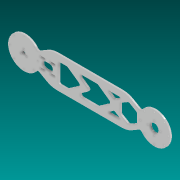
# Autodesk Inventor part: arm1v2
Saved by Autodesk Inventor 2020.3 (Build 243373000, 373)
## iProperties
Created: 2020-05-23
Part Number: arm1v2
Material: Aluminum 6061
Document SubType Name: Sheet Metal
Designer: Svend
Mass: 232.394 g
Surface Area: 513.63 cm^2
Volume: 86.0718 cm^3
Density: 2.7 g/cm^3
Sheet Metal Rule: Default_mm
Appearance: Aluminum - Polished
Author: Svend
Autodesk Inventor part; units mm, degrees
ref_plane "YZ Plane" through (0, 0, 0) normal (1, 0, 0) x (0, 1, 0)
ref_plane "XZ Plane" through (0, 0, 0) normal (0, 1, 0) x (-1, 0, 0)
ref_plane "XY Plane" through (0, 0, 0) normal (0, 0, 1) x (1, 0, 0)
sketch "Sketch1" plane through (0, 0, 0) normal (0, 0, 1) x (1, 0, 0)
  circle A0 centre (346.3464, 0) radius 1.55
  circle A1 centre (330.346, 0) radius 11
  arc A2 (52.2721, 10.7279) -> (52.2721, 14.7279) centre (52.2721, 12.7279) ccw
  line L0 (52.2721, 10.7279) -> (42.2721, 10.7279)
  arc A3 (42.2721, 14.7279) -> (42.2721, 10.7279) centre (42.2721, 12.7279) ccw
  line L1 (42.2721, 14.7279) -> (52.2721, 14.7279)
  arc A4 (77.7279, 10.7279) -> (77.7279, 14.7279) centre (77.7279, 12.7279) ccw
  line L2 (77.7279, 10.7279) -> (67.7279, 10.7279)
  arc A5 (67.7279, 14.7279) -> (67.7279, 10.7279) centre (67.7279, 12.7279) ccw
  line L3 (67.7279, 14.7279) -> (77.7279, 14.7279)
  arc A6 (52.2721, -14.7279) -> (52.2721, -10.7279) centre (52.2721, -12.7279) ccw
  line L4 (52.2721, -14.7279) -> (42.2721, -14.7279)
  arc A7 (42.2721, -10.7279) -> (42.2721, -14.7279) centre (42.2721, -12.7279) ccw
  line L5 (42.2721, -10.7279) -> (52.2721, -10.7279)
  arc A8 (67.7279, -10.7279) -> (67.7279, -14.7279) centre (67.7279, -12.7279) ccw
  line L6 (67.7279, -10.7279) -> (77.7279, -10.7279)
  arc A9 (77.7279, -14.7279) -> (77.7279, -10.7279) centre (77.7279, -12.7279) ccw
  line L7 (77.7279, -14.7279) -> (67.7279, -14.7279)
  circle A10 centre (60, 0) radius 8.5
  circle A11 centre (28, 0) radius 0.5
  line L8 (0, -40) -> (330.346, -40)
  arc A12 (330.346, -40) -> (330.346, 40) centre (330.346, 0) ccw
  line L9 (330.346, 40) -> (0, 40)
  arc A13 (0, 40) -> (0, -40) centre (0, 0) ccw
  line L10 (-4.8, -1) -> (-4.8, 1)
  line L11 (-4.8, 1) -> (-3.873, 1)
  arc A14 (-3.873, -1) -> (-3.873, 1) centre (0, 0) ccw
  line L12 (-3.873, -1) -> (-4.8, -1)
  circle A15 centre (0, 8) radius 2
  circle A16 centre (-6.9282, -4) radius 2
  circle A17 centre (6.9282, -4) radius 2
  circle A18 centre (19.799, 19.799) radius 0.5
  circle A19 centre (0, 28) radius 0.5
  circle A20 centre (-19.799, 19.799) radius 0.5
  circle A21 centre (-28, 0) radius 0.5
  circle A22 centre (-19.799, -19.799) radius 0.5
  circle A23 centre (0, -28) radius 0.5
  circle A24 centre (19.799, -19.799) radius 0.5
  circle A25 centre (330.346, 16.0004) radius 1.55
  circle A26 centre (314.3456, 0) radius 1.55
  circle A27 centre (330.346, -16.0004) radius 1.55
  line L13 (55, 0) -> (65, 0) construction
  line L14 (55, -8.5) -> (65, -8.5)
  line L15 (65, 8.5) -> (55, 8.5)
  arc A28 (55, 8.5) -> (55, -8.5) centre (55, 0) ccw
  arc A29 (65, -8.5) -> (65, 8.5) centre (65, 0) ccw
  point P0 (-4.8, 0)
  point P1 (4, 0)
  point P2 (370.346, 0)
  dimension "d0" = 4
  dimension "d1" = 8.8
  dimension "d2" = 2
  dimension "d6" = 4
  dimension "d7" = 8
  dimension "d14" = 360
  dimension "d16" = 28
  dimension "d17" = 1
  dimension "d20" = 360
  dimension "d22" = 17
  dimension "d23" = 60
  dimension "d24" = 2
  dimension "d25" = 10
  dimension "d26" = 12.7279
  dimension "d27" = 17.7279
  dimension "d28" = 12.7279
  dimension "d29" = 17.7279
  dimension "d30" = 17.7279
  dimension "d31" = 17.7279
  dimension "d32" = 22
  dimension "d33" = 39.9999
  dimension "d35" = 3.1
  dimension "d36" = 16.0004
  dimension "d39" = 360
  dimension "d72" = 270.346
  dimension "d87" = 5
  measures "d0" radius of A14
  measures "d1" distance from line of point (4, 0) L10
  measures "d2" distance between parallel lines of L12 L11
  measures "d6" diameter of A15
  measures "d7" distance of A14.centre A15.centre
  measures "d16" distance of A14.centre A11.centre
  measures "d17" diameter of A11
  measures "d22" diameter of A10
  measures "d23" distance of A14.centre A10.centre
  measures "d24" radius of A3
  measures "d25" distance of L0.start L0.end
  measures "d26" vertical distance of A10.centre A2.centre
  measures "d27" horizontal distance of A10.centre A3.centre
  measures "d28" vertical distance of A8.centre A10.centre
  measures "d29" horizontal distance of A9.centre A10.centre
  measures "d30" horizontal distance of A7.centre A10.centre
  measures "d31" horizontal distance of A4.centre A10.centre
  measures "d32" diameter of A1
  measures "d33" radius of A13
  measures "d35" diameter of A0
  measures "d36" distance of A1.centre A0.centre
  measures "d72" distance of A1.centre A10.centre
  measures "d87" distance of A10.centre L13.end
extrude "Plate1" add sketch "Sketch1" along normal mid plane 4 contours A11 | A13 L9 A12 L8 | A18 | A19 | A20 | A21 | A22 | A23 | A24
sketch "Sketch2" plane through (0, 0, -2) normal (0, 0, -1) x (-1, 0, 0)
  circle A0 centre (-330.346, 0) radius 11 projected
  line L0 (-77.7279, -10.7279) -> (-67.7279, -10.7279) projected
  arc A1 (-67.7279, -14.7279) -> (-67.7279, -10.7279) centre (-67.7279, -12.7279) ccw projected
  line L1 (-67.7279, -14.7279) -> (-77.7279, -14.7279) projected
  arc A2 (-77.7279, -10.7279) -> (-77.7279, -14.7279) centre (-77.7279, -12.7279) ccw projected
  line L2 (-42.2721, -14.7279) -> (-52.2721, -14.7279) projected
  arc A3 (-52.2721, -10.7279) -> (-52.2721, -14.7279) centre (-52.2721, -12.7279) ccw projected
  line L3 (-52.2721, -10.7279) -> (-42.2721, -10.7279) projected
  arc A4 (-42.2721, -14.7279) -> (-42.2721, -10.7279) centre (-42.2721, -12.7279) ccw projected
  line L4 (-67.7279, 10.7279) -> (-77.7279, 10.7279) projected
  arc A5 (-77.7279, 14.7279) -> (-77.7279, 10.7279) centre (-77.7279, 12.7279) ccw projected
  line L5 (-77.7279, 14.7279) -> (-67.7279, 14.7279) projected
  arc A6 (-67.7279, 10.7279) -> (-67.7279, 14.7279) centre (-67.7279, 12.7279) ccw projected
  line L6 (-42.2721, 10.7279) -> (-52.2721, 10.7279) projected
  arc A7 (-52.2721, 14.7279) -> (-52.2721, 10.7279) centre (-52.2721, 12.7279) ccw projected
  line L7 (-52.2721, 14.7279) -> (-42.2721, 14.7279) projected
  arc A8 (-42.2721, 10.7279) -> (-42.2721, 14.7279) centre (-42.2721, 12.7279) ccw projected
  line L8 (3.873, 1) -> (4.8, 1) projected
  line L9 (4.8, 1) -> (4.8, -1) projected
  line L10 (4.8, -1) -> (3.873, -1) projected
  arc A9 (3.873, 1) -> (3.873, -1) centre (0, 0) ccw projected
  circle A10 centre (-6.9282, -4) radius 2 projected
  circle A11 centre (6.9282, -4) radius 2 projected
  circle A12 centre (0, 8) radius 2 projected
  circle A13 centre (-330.346, -16.0004) radius 1.55 projected
  circle A14 centre (-314.3456, 0) radius 1.55 projected
  circle A15 centre (-330.346, 16.0004) radius 1.55 projected
  circle A16 centre (-346.3464, 0) radius 1.55 projected
  line L11 (0, -40) -> (-330.346, -40) projected
  arc A17 (0, -40) -> (0, 40) centre (0, 0) ccw projected
  line L12 (-330.346, 40) -> (0, 40) projected
  arc A18 (-330.346, 40) -> (-330.346, -40) centre (-330.346, 0) ccw projected
  line L13 (-330.346, 40) -> (0, 40) projected
  arc A19 (-330.346, 40) -> (-330.346, -40) centre (-330.346, 0) ccw projected
  line L14 (-330.346, 0) -> (0, 0)
  line L15 (0, -40) -> (-330.346, -40) projected
  line L16 (-210.2693, -25) -> (-250.2693, -25)
  line L17 (-250.2693, -25) -> (-228.346, -12.3426)
  line L18 (-228.346, -12.3426) -> (-210.2693, -25)
  line L19 (-261.064, -40) -> (-295.705, -20)
  line L20 (-222.346, 0) -> (-186.6423, -25)
  line L21 (-186.6423, -25) -> (-131.6423, -25)
  line L22 (-131.6423, -25) -> (-167.346, 0)
  line L23 (-109.6423, -25) -> (-145.346, 0)
  line L24 (-87.346, -25) -> (-109.6423, -25)
  line L25 (-87.346, -25) -> (-87.346, 0)
  line L26 (-210.2693, 25) -> (-250.2693, 25)
  line L27 (-250.2693, 25) -> (-228.346, 12.3426)
  line L28 (-228.346, 12.3426) -> (-210.2693, 25)
  line L29 (-222.346, 0) -> (-186.6423, 25)
  line L30 (-186.6423, 25) -> (-131.6423, 25)
  line L31 (-131.6423, 25) -> (-167.346, 0)
  line L32 (-109.6423, 25) -> (-145.346, 0)
  line L33 (-87.346, 25) -> (-109.6423, 25)
  line L34 (-87.346, 25) -> (-87.346, 0)
  line L35 (-295.705, 20) -> (-261.064, 40)
  line L36 (-261.064, 40) -> (-330.346, 40)
  arc A20 (-295.705, 20) -> (-330.346, 40) centre (-330.346, 0) ccw
  arc A21 (-330.346, -40) -> (-295.705, -20) centre (-330.346, 0) ccw
  line L37 (-286.9966, -12.5) -> (-286.9966, 12.5)
  line L38 (-286.9966, 12.5) -> (-265.346, 25)
  line L39 (-265.346, 25) -> (-243.6954, 12.5)
  line L40 (-243.6954, 12.5) -> (-243.6954, -12.5)
  line L41 (-243.6954, -12.5) -> (-265.346, -25)
  line L42 (-265.346, -25) -> (-286.9966, -12.5)
  line L43 (-165.173, 40) -> (-165.173, -40)
  line L44 (0, 40) -> (-330.346, 40)
  line L45 (-69.282, -40) -> (-34.641, -20)
  arc A22 (-34.641, -20) -> (0, -40) centre (0, 0) ccw
  line L46 (-330.346, -40) -> (0, -40) projected
  line L47 (0, -40) -> (-69.282, -40)
  line L48 (-69.282, 40) -> (-34.641, 20)
  arc A23 (0, 40) -> (-34.641, 20) centre (0, 0) ccw
  line L49 (0, 40) -> (-69.282, 40)
  point P0 (-323.7858, 40)
  point P1 (-323.7858, -40)
  point P2 (-265.346, 0)
  point P3 (-228.346, 0)
  point P4 (-265.346, 0)
  dimension "d47" = 40
  dimension "d49" = 102
  dimension "d52" = 35
  dimension "d54" = 55
  dimension "d55" = 25
  dimension "d59" = 108
  dimension "d60" = 185
  dimension "d64" = 58
  dimension "d67" = 65
  constraints: 69 end point, 15 symmetric about line, 9 parallel, 9 point on line, 8 point on circle, 4 centre point, 4 collinear, 4 horizontal alignment, 4 line through centre, 3 coincident, 3 horizontal, 3 midpoint, 3 perpendicular, 3 tangent, 1 vertical alignment, 15 other
  measures "d47" distance of L16.start L16.end
  measures "d49" distance of A0.centre point (-228.346, 0)
  measures "d52" angle of L22 L21
  measures "d54" distance of L20.end L21.end
  measures "d55" distance between parallel lines of L14 L21
  measures "d59" distance of A0.centre L20.start
  measures "d60" distance of A0.centre L23.end
  measures "d64" distance from line of L25 L23.end
  measures "d67" distance of A0.centre point (-265.346, 0)
extrude "Cut1" cut sketch "Sketch2" against normal blind 4 contours L11 L45 A22 | A23 L48 L12 | L11 A21 L19 | L43 L22 L21 | L21 L20 L14 L22 L43 | L35 A20 L12 | L43 L31 L14 L29 L30 | L30 L31 L43 | L32 L33 L34 L14 | L14 L25 L24 L23 | L37 L38 L39 L40 L14 | L14 L40 L41 L42 L37 | L16 L17 L18 | L28 L27 L26
fillet "Fillet1" radius 2 6 edges at (250.2693, -25, 0) (210.2693, -25, 0) (228.346, -12.3426, 0) (250.2693, 25, 0) (228.346, 12.3426, 0) (210.2693, 25, 0)
fillet "Fillet2" radius 5 6 edges at (286.9966, -12.5, 0) (265.346, -25, 0) (243.6954, -12.5, 0) (243.6954, 12.5, 0) (265.346, 25, 0) (286.9966, 12.5, 0)
fillet "Fillet3" radius 5 11 edges at (222.346, 0, 0) (186.6423, -25, 0) (131.6423, -25, 0) (131.6423, 25, 0) (167.346, 0, 0) (186.6423, 25, 0) (145.346, 0, 0) (109.6423, -25, 0) (87.346, -25, 0) (87.346, 25, 0) (109.6423, 25, 0)
fillet "Fillet4" radius 50 4 edges at (261.064, -40, 0) (261.064, 40, 0) (69.282, 40, 0) (69.282, -40, 0)
fillet "Fillet5" radius 5 4 edges at (295.705, -20, 0) (295.705, 20, 0) (34.641, -20, 0) (34.641, 20, 0)
sketch "Sketch3" plane through (0, 0, -2) normal (0, 0, -1) x (-1, 0, 0)
  arc A0 (-82.6794, -40) -> (-57.6794, -33.3012) centre (-82.6794, 10) ccw projected
  line L0 (-57.6794, -33.3012) -> (-38.7298, -22.3607) projected
  arc A1 (-32.2043, -23.7251) -> (-38.7298, -22.3607) centre (-36.2298, -26.6908) ccw projected
  arc A2 (-32.2043, -23.7251) -> (-32.2043, 23.7251) centre (0, 0) ccw projected
  arc A3 (-38.7298, 22.3607) -> (-32.2043, 23.7251) centre (-36.2298, 26.6908) ccw projected
  line L1 (-38.7298, 22.3607) -> (-57.6794, 33.3012) projected
  arc A4 (-57.6794, 33.3012) -> (-82.6794, 40) centre (-82.6794, -10) ccw projected
  line L2 (-247.6666, 40) -> (-82.6794, 40) projected
  arc A5 (-247.6666, 40) -> (-272.6666, 33.3012) centre (-247.6666, -10) ccw projected
  line L3 (-272.6666, 33.3012) -> (-291.6162, 22.3607) projected
  arc A6 (-298.1417, 23.7251) -> (-291.6162, 22.3607) centre (-294.1162, 26.6908) ccw projected
  arc A7 (-298.1417, 23.7251) -> (-298.1417, -23.7251) centre (-330.346, 0) ccw projected
  arc A8 (-291.6162, -22.3607) -> (-298.1417, -23.7251) centre (-294.1162, -26.6908) ccw projected
  line L4 (-291.6162, -22.3607) -> (-272.6666, -33.3012) projected
  arc A9 (-272.6666, -33.3012) -> (-247.6666, -40) centre (-247.6666, 10) ccw projected
  line L5 (-82.6794, -40) -> (-247.6666, -40) projected
  arc A10 (-161.4966, 4.0958) -> (-161.4966, -4.0958) centre (-158.6288, 0) ccw projected
  line L6 (-161.4966, -4.0958) -> (-144.6324, -15.9042) projected
  arc A11 (-147.5003, -25) -> (-144.6324, -15.9042) centre (-147.5003, -20) ccw projected
  line L7 (-147.5003, -25) -> (-185.0658, -25) projected
  arc A12 (-187.9337, -24.0958) -> (-185.0658, -25) centre (-185.0658, -20) ccw projected
  line L8 (-187.9337, -24.0958) -> (-216.4966, -4.0958) projected
  arc A13 (-216.4966, 4.0958) -> (-216.4966, -4.0958) centre (-213.6288, 0) ccw projected
  line L9 (-216.4966, 4.0958) -> (-187.9337, 24.0958) projected
  arc A14 (-185.0658, 25) -> (-187.9337, 24.0958) centre (-185.0658, 20) ccw projected
  line L10 (-185.0658, 25) -> (-147.5003, 25) projected
  arc A15 (-144.6324, 15.9042) -> (-147.5003, 25) centre (-147.5003, 20) ccw projected
  line L11 (-144.6324, 15.9042) -> (-161.4966, 4.0958) projected
  line L12 (-215.4654, 21.3617) -> (-227.3023, 13.0734) projected
  arc A16 (-229.4494, 12.9796) -> (-227.3023, 13.0734) centre (-228.4494, 14.7117) ccw projected
  line L13 (-229.4494, 12.9796) -> (-243.8052, 21.2679) projected
  arc A17 (-242.8052, 25) -> (-243.8052, 21.2679) centre (-242.8052, 23) ccw projected
  line L14 (-242.8052, 25) -> (-216.6125, 25) projected
  arc A18 (-215.4654, 21.3617) -> (-216.6125, 25) centre (-216.6125, 23) ccw projected
  line L15 (-227.3023, -13.0734) -> (-215.4654, -21.3617) projected
  arc A19 (-216.6125, -25) -> (-215.4654, -21.3617) centre (-216.6125, -23) ccw projected
  line L16 (-216.6125, -25) -> (-242.8052, -25) projected
  arc A20 (-243.8052, -21.2679) -> (-242.8052, -25) centre (-242.8052, -23) ccw projected
  line L17 (-243.8052, -21.2679) -> (-229.4494, -12.9796) projected
  arc A21 (-227.3023, -13.0734) -> (-229.4494, -12.9796) centre (-228.4494, -14.7117) ccw projected
  line L18 (-267.846, -23.5566) -> (-284.4966, -13.9434) projected
  arc A22 (-286.9966, -9.6132) -> (-284.4966, -13.9434) centre (-281.9966, -9.6132) ccw projected
  line L19 (-286.9966, -9.6132) -> (-286.9966, 9.6132) projected
  arc A23 (-284.4966, 13.9434) -> (-286.9966, 9.6132) centre (-281.9966, 9.6132) ccw projected
  line L20 (-284.4966, 13.9434) -> (-267.846, 23.5566) projected
  arc A24 (-262.846, 23.5566) -> (-267.846, 23.5566) centre (-265.346, 19.2265) ccw projected
  line L21 (-262.846, 23.5566) -> (-246.1954, 13.9434) projected
  arc A25 (-243.6954, 9.6132) -> (-246.1954, 13.9434) centre (-248.6954, 9.6132) ccw projected
  line L22 (-243.6954, 9.6132) -> (-243.6954, -9.6132) projected
  arc A26 (-246.1954, -13.9434) -> (-243.6954, -9.6132) centre (-248.6954, -9.6132) ccw projected
  line L23 (-246.1954, -13.9434) -> (-262.846, -23.5566) projected
  arc A27 (-267.846, -23.5566) -> (-262.846, -23.5566) centre (-265.346, -19.2265) ccw projected
  line L24 (-92.346, -25) -> (-108.0658, -25) projected
  arc A28 (-110.9337, -24.0958) -> (-108.0658, -25) centre (-108.0658, -20) ccw projected
  line L25 (-110.9337, -24.0958) -> (-139.4966, -4.0958) projected
  arc A29 (-139.4966, 4.0958) -> (-139.4966, -4.0958) centre (-136.6288, 0) ccw projected
  line L26 (-139.4966, 4.0958) -> (-110.9337, 24.0958) projected
  arc A30 (-108.0658, 25) -> (-110.9337, 24.0958) centre (-108.0658, 20) ccw projected
  line L27 (-108.0658, 25) -> (-92.346, 25) projected
  arc A31 (-87.346, 20) -> (-92.346, 25) centre (-92.346, 20) ccw projected
  line L28 (-87.346, 20) -> (-87.346, -20) projected
  arc A32 (-92.346, -25) -> (-87.346, -20) centre (-92.346, -20) ccw projected
  circle A33 centre (-330.346, 0) radius 11 projected
  line L29 (-77.7279, -10.7279) -> (-67.7279, -10.7279) projected
  arc A34 (-67.7279, -14.7279) -> (-67.7279, -10.7279) centre (-67.7279, -12.7279) ccw projected
  line L30 (-67.7279, -14.7279) -> (-77.7279, -14.7279) projected
  arc A35 (-77.7279, -10.7279) -> (-77.7279, -14.7279) centre (-77.7279, -12.7279) ccw projected
  line L31 (-42.2721, -14.7279) -> (-52.2721, -14.7279) projected
  arc A36 (-52.2721, -10.7279) -> (-52.2721, -14.7279) centre (-52.2721, -12.7279) ccw projected
  line L32 (-52.2721, -10.7279) -> (-42.2721, -10.7279) projected
  arc A37 (-42.2721, -14.7279) -> (-42.2721, -10.7279) centre (-42.2721, -12.7279) ccw projected
  line L33 (-67.7279, 10.7279) -> (-77.7279, 10.7279) projected
  arc A38 (-77.7279, 14.7279) -> (-77.7279, 10.7279) centre (-77.7279, 12.7279) ccw projected
  line L34 (-77.7279, 14.7279) -> (-67.7279, 14.7279) projected
  arc A39 (-67.7279, 10.7279) -> (-67.7279, 14.7279) centre (-67.7279, 12.7279) ccw projected
  line L35 (-42.2721, 10.7279) -> (-52.2721, 10.7279) projected
  arc A40 (-52.2721, 14.7279) -> (-52.2721, 10.7279) centre (-52.2721, 12.7279) ccw projected
  line L36 (-52.2721, 14.7279) -> (-42.2721, 14.7279) projected
  arc A41 (-42.2721, 10.7279) -> (-42.2721, 14.7279) centre (-42.2721, 12.7279) ccw projected
  line L37 (3.873, 1) -> (4.8, 1) projected
  line L38 (4.8, 1) -> (4.8, -1) projected
  line L39 (4.8, -1) -> (3.873, -1) projected
  arc A42 (3.873, 1) -> (3.873, -1) centre (0, 0) ccw projected
  circle A43 centre (-6.9282, -4) radius 2 projected
  circle A44 centre (6.9282, -4) radius 2 projected
  circle A45 centre (0, 8) radius 2 projected
  circle A46 centre (-330.346, -16.0004) radius 1.55 projected
  circle A47 centre (-314.3456, 0) radius 1.55 projected
  circle A48 centre (-330.346, 16.0004) radius 1.55 projected
  circle A49 centre (-346.3464, 0) radius 1.55 projected
  circle A50 centre (-365.846, 0) radius 1.5
  circle A51 centre (-355.4483, -25.1023) radius 1.5
  circle A52 centre (-330.346, -35.5) radius 1.5
  circle A53 centre (-305.2437, -25.1023) radius 1.5
  circle A54 centre (-294.846, 0) radius 1.5
  circle A55 centre (-305.2437, 25.1023) radius 1.5
  circle A56 centre (-330.346, 35.5) radius 1.5
  circle A57 centre (-355.4483, 25.1023) radius 1.5
  point P0 (0, 0)
  dimension "d73" = 3
  dimension "d74" = 35.5
  dimension "d77" = 360
  constraints: 8 centre point, 1 horizontal alignment, 17 other
  measures "d73" diameter of A50
  measures "d74" distance of A33.centre A50.centre
extrude "Cut2" cut sketch "Sketch3" against normal blind 4 contours A50 | A51 | A52 | A53 | A54 | A55 | A56 | A57
chamfer "Chamfer2" distance 1.5 angle 45 4 edges at (344.7964, 0, -2) (328.796, 16.0004, -2) (312.7956, 0, -2) (328.796, -16.0004, -2)
sketch "Sketch4" plane through (0, 0, 2) normal (0, 0, 1) x (1, 0, 0)
  circle A0 centre (314.3456, 0) radius 3.05 projected
  circle A1 centre (346.3464, 0) radius 3.05 projected
  circle A2 centre (330.346, 35.5) radius 1.5 projected
  circle A3 centre (294.846, 0) radius 1.5 projected
  circle A4 centre (330.346, -35.5) radius 1.5 projected
  circle A5 centre (365.846, 0) radius 1.5 projected
  circle A6 centre (355.4483, -25.1023) radius 1.5 projected
  circle A7 centre (305.2437, -25.1023) radius 1.5 projected
  circle A8 centre (305.2437, 25.1023) radius 1.5 projected
  circle A9 centre (355.4483, 25.1023) radius 1.5 projected
  arc A10 (57.6794, -33.3012) -> (82.6794, -40) centre (82.6794, 10) ccw projected
  line L0 (57.6794, -33.3012) -> (38.7298, -22.3607) projected
  arc A11 (38.7298, -22.3607) -> (32.2043, -23.7251) centre (36.2298, -26.6908) ccw projected
  arc A12 (32.2043, 23.7251) -> (32.2043, -23.7251) centre (0, 0) ccw projected
  arc A13 (32.2043, 23.7251) -> (38.7298, 22.3607) centre (36.2298, 26.6908) ccw projected
  line L1 (38.7298, 22.3607) -> (57.6794, 33.3012) projected
  arc A14 (82.6794, 40) -> (57.6794, 33.3012) centre (82.6794, -10) ccw projected
  line L2 (247.6666, 40) -> (82.6794, 40) projected
  arc A15 (272.6666, 33.3012) -> (247.6666, 40) centre (247.6666, -10) ccw projected
  line L3 (272.6666, 33.3012) -> (291.6162, 22.3607) projected
  arc A16 (291.6162, 22.3607) -> (298.1417, 23.7251) centre (294.1162, 26.6908) ccw projected
  arc A17 (298.1417, -23.7251) -> (298.1417, 23.7251) centre (330.346, 0) ccw projected
  arc A18 (298.1417, -23.7251) -> (291.6162, -22.3607) centre (294.1162, -26.6908) ccw projected
  line L4 (291.6162, -22.3607) -> (272.6666, -33.3012) projected
  arc A19 (247.6666, -40) -> (272.6666, -33.3012) centre (247.6666, 10) ccw projected
  line L5 (82.6794, -40) -> (247.6666, -40) projected
  arc A20 (161.4966, -4.0958) -> (161.4966, 4.0958) centre (158.6288, 0) ccw projected
  line L6 (161.4966, -4.0958) -> (144.6324, -15.9042) projected
  arc A21 (144.6324, -15.9042) -> (147.5003, -25) centre (147.5003, -20) ccw projected
  line L7 (147.5003, -25) -> (185.0658, -25) projected
  arc A22 (185.0658, -25) -> (187.9337, -24.0958) centre (185.0658, -20) ccw projected
  line L8 (187.9337, -24.0958) -> (216.4966, -4.0958) projected
  arc A23 (216.4966, -4.0958) -> (216.4966, 4.0958) centre (213.6288, 0) ccw projected
  line L9 (216.4966, 4.0958) -> (187.9337, 24.0958) projected
  arc A24 (187.9337, 24.0958) -> (185.0658, 25) centre (185.0658, 20) ccw projected
  line L10 (185.0658, 25) -> (147.5003, 25) projected
  arc A25 (147.5003, 25) -> (144.6324, 15.9042) centre (147.5003, 20) ccw projected
  line L11 (144.6324, 15.9042) -> (161.4966, 4.0958) projected
  line L12 (215.4654, 21.3617) -> (227.3023, 13.0734) projected
  arc A26 (227.3023, 13.0734) -> (229.4494, 12.9796) centre (228.4494, 14.7117) ccw projected
  line L13 (229.4494, 12.9796) -> (243.8052, 21.2679) projected
  arc A27 (243.8052, 21.2679) -> (242.8052, 25) centre (242.8052, 23) ccw projected
  line L14 (242.8052, 25) -> (216.6125, 25) projected
  arc A28 (216.6125, 25) -> (215.4654, 21.3617) centre (216.6125, 23) ccw projected
  line L15 (227.3023, -13.0734) -> (215.4654, -21.3617) projected
  arc A29 (215.4654, -21.3617) -> (216.6125, -25) centre (216.6125, -23) ccw projected
  line L16 (216.6125, -25) -> (242.8052, -25) projected
  arc A30 (242.8052, -25) -> (243.8052, -21.2679) centre (242.8052, -23) ccw projected
  line L17 (243.8052, -21.2679) -> (229.4494, -12.9796) projected
  arc A31 (229.4494, -12.9796) -> (227.3023, -13.0734) centre (228.4494, -14.7117) ccw projected
  line L18 (267.846, -23.5566) -> (284.4966, -13.9434) projected
  arc A32 (284.4966, -13.9434) -> (286.9966, -9.6132) centre (281.9966, -9.6132) ccw projected
  line L19 (286.9966, -9.6132) -> (286.9966, 9.6132) projected
  arc A33 (286.9966, 9.6132) -> (284.4966, 13.9434) centre (281.9966, 9.6132) ccw projected
  line L20 (284.4966, 13.9434) -> (267.846, 23.5566) projected
  arc A34 (267.846, 23.5566) -> (262.846, 23.5566) centre (265.346, 19.2265) ccw projected
  line L21 (262.846, 23.5566) -> (246.1954, 13.9434) projected
  arc A35 (246.1954, 13.9434) -> (243.6954, 9.6132) centre (248.6954, 9.6132) ccw projected
  line L22 (243.6954, 9.6132) -> (243.6954, -9.6132) projected
  arc A36 (243.6954, -9.6132) -> (246.1954, -13.9434) centre (248.6954, -9.6132) ccw projected
  line L23 (246.1954, -13.9434) -> (262.846, -23.5566) projected
  arc A37 (262.846, -23.5566) -> (267.846, -23.5566) centre (265.346, -19.2265) ccw projected
  line L24 (92.346, -25) -> (108.0658, -25) projected
  arc A38 (108.0658, -25) -> (110.9337, -24.0958) centre (108.0658, -20) ccw projected
  line L25 (110.9337, -24.0958) -> (139.4966, -4.0958) projected
  arc A39 (139.4966, -4.0958) -> (139.4966, 4.0958) centre (136.6288, 0) ccw projected
  line L26 (139.4966, 4.0958) -> (110.9337, 24.0958) projected
  arc A40 (110.9337, 24.0958) -> (108.0658, 25) centre (108.0658, 20) ccw projected
  line L27 (108.0658, 25) -> (92.346, 25) projected
  arc A41 (92.346, 25) -> (87.346, 20) centre (92.346, 20) ccw projected
  line L28 (87.346, 20) -> (87.346, -20) projected
  arc A42 (87.346, -20) -> (92.346, -25) centre (92.346, -20) ccw projected
  arc A43 (55, 8.5) -> (55, -8.5) centre (55, 0) ccw projected
  line L29 (55, -8.5) -> (65, -8.5) projected
  arc A44 (65, -8.5) -> (65, 8.5) centre (65, 0) ccw projected
  line L30 (65, 8.5) -> (55, 8.5) projected
  circle A45 centre (330.346, 0) radius 11 projected
  line L31 (77.7279, -10.7279) -> (67.7279, -10.7279) projected
  arc A46 (67.7279, -10.7279) -> (67.7279, -14.7279) centre (67.7279, -12.7279) ccw projected
  line L32 (67.7279, -14.7279) -> (77.7279, -14.7279) projected
  arc A47 (77.7279, -14.7279) -> (77.7279, -10.7279) centre (77.7279, -12.7279) ccw projected
  line L33 (42.2721, -14.7279) -> (52.2721, -14.7279) projected
  arc A48 (52.2721, -14.7279) -> (52.2721, -10.7279) centre (52.2721, -12.7279) ccw projected
  line L34 (52.2721, -10.7279) -> (42.2721, -10.7279) projected
  arc A49 (42.2721, -10.7279) -> (42.2721, -14.7279) centre (42.2721, -12.7279) ccw projected
  line L35 (67.7279, 10.7279) -> (77.7279, 10.7279) projected
  arc A50 (77.7279, 10.7279) -> (77.7279, 14.7279) centre (77.7279, 12.7279) ccw projected
  line L36 (77.7279, 14.7279) -> (67.7279, 14.7279) projected
  arc A51 (67.7279, 14.7279) -> (67.7279, 10.7279) centre (67.7279, 12.7279) ccw projected
  line L37 (42.2721, 10.7279) -> (52.2721, 10.7279) projected
  arc A52 (52.2721, 10.7279) -> (52.2721, 14.7279) centre (52.2721, 12.7279) ccw projected
  line L38 (52.2721, 14.7279) -> (42.2721, 14.7279) projected
  arc A53 (42.2721, 14.7279) -> (42.2721, 10.7279) centre (42.2721, 12.7279) ccw projected
  line L39 (-3.873, 1) -> (-4.8, 1) projected
  line L40 (-4.8, 1) -> (-4.8, -1) projected
  line L41 (-4.8, -1) -> (-3.873, -1) projected
  arc A54 (-3.873, -1) -> (-3.873, 1) centre (0, 0) ccw projected
  circle A55 centre (6.9282, -4) radius 2 projected
  circle A56 centre (-6.9282, -4) radius 2 projected
  circle A57 centre (0, 8) radius 2 projected
  circle A58 centre (330.346, 16.0004) radius 3.05 projected
  circle A59 centre (330.346, -16.0004) radius 3.05 projected
  point P0 (0, 0)
  point P1 (35.5, 0)
  point P2 (25.1023, 25.1023)
  point P3 (0, 35.5)
  point P4 (-25.1023, 25.1023)
  point P5 (-35.5, 0)
  point P6 (-25.1023, -25.1023)
  point P7 (0, -35.5)
  point P8 (25.1023, -25.1023)
  dimension "d88" = 35.5
  dimension "d91" = 360
  constraints: 1 horizontal alignment, 9 other
  measures "d88" distance of A54.centre point (35.5, 0)
hole "Hole1" at (0, -35.5, 2) at (-25.1023, -25.1023, 2) at (-35.5, 0, 2) at (-25.1023, 25.1023, 2) at (0, 35.5, 2) at (25.1023, 25.1023, 2) at (35.5, 0, 2) at (25.1023, -25.1023, 2) direction (0, 0, -1) diameter 2.459 depth 8.8 tip angle 118 thread size "M3x0.5" class "6H" standard "ISO Metric profile"
equation "\"d41\" = Thickness"
equation "\"BendRadius\" = Thickness"
equation "\"BendReliefWidth\" = Thickness"
equation "\"BendReliefDepth\" = 0.5 * Thickness"
equation "\"CornerReliefSize\" = 4 * Thickness"
equation "\"MinimumRemnant\" = 2 * Thickness"
equation "\"TransitionRadius\" = BendRadius"
equation "\"JacobiRadiusSize\" = BendRadius"
equation "\"GapSize\" = Thickness"
equation "\"Thickness\" = 4"
body "Solid1"
